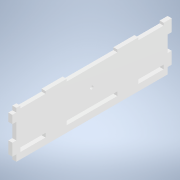
# Autodesk Inventor part: case top sides
Saved by Autodesk Inventor 2022 (Build 260153000, 153)
## iProperties
Created: 2021-05-28
Part Number: case top sides
Material: ABS Plastic
Document SubType Name: Modeling
Designer: benka
Density: 1.06 g/cm^3
Appearance: Smooth - White
Author: benka
Autodesk Inventor part; units mm, degrees
ref_plane "YZ Plane" through (0, 0, 0) normal (1, 0, 0) x (0, 1, 0)
ref_plane "XZ Plane" through (0, 0, 0) normal (0, 1, 0) x (-1, 0, 0)
ref_plane "XY Plane" through (0, 0, 0) normal (0, 0, 1) x (1, 0, 0)
sketch "Sketch1" plane through (0, 0, 0) normal (1, 0, 0) x (0, 1, 0)
  circle A0 centre (0, 0) radius 2
  line L0 (-20.007, 88.601) -> (-20.007, 57.351) projected
  line L1 (-20.007, 57.351) -> (-25.007, 57.351) projected
  line L2 (-25.007, 88.601) -> (-25.007, 57.351) projected
  line L3 (-20.007, 88.601) -> (-25.007, 88.601) projected
  line L4 (-20.007, 31.101) -> (-20.007, -31.899) projected
  line L5 (-20.007, -31.899) -> (-25.007, -31.899) projected
  line L6 (-25.007, 31.101) -> (-25.007, -31.899) projected
  line L7 (-20.007, 31.101) -> (-25.007, 31.101) projected
  line L8 (-20.007, -58.149) -> (-20.007, -89.399) projected
  line L9 (-20.007, -89.399) -> (-25.007, -89.399) projected
  line L10 (-25.007, -58.149) -> (-25.007, -89.399) projected
  line L11 (-20.007, -58.149) -> (-25.007, -58.149) projected
  line L12 (19.993, 93.601) -> (19.993, 98.601)
  line L13 (19.993, 98.601) -> (9.9915, 98.601) projected
  line L14 (9.9915, 93.601) -> (9.9915, 98.601) projected
  line L15 (-10.0085, 93.601) -> (-10.0085, 98.601) projected
  line L16 (-25.0077, 98.601) -> (-10.0085, 98.601) projected
  line L17 (-25.007, 93.601) -> (-25.007, 98.601) projected
  line L18 (-25.007, 93.601) -> (-33.007, 93.601)
  line L19 (-33.007, 93.601) -> (-33.007, -94.399)
  line L20 (-10.0085, 93.601) -> (9.9915, 93.601)
  line L21 (24.993, -99.399) -> (24.993, -94.399)
  line L22 (9.993, -99.399) -> (24.993, -99.399) projected
  line L23 (9.993, -99.399) -> (9.993, -94.399) projected
  line L24 (-10.0077, -94.399) -> (9.993, -94.399) projected
  line L25 (-10.0077, -99.399) -> (-10.0077, -94.399) projected
  line L26 (-25.0077, -99.399) -> (-10.0077, -99.399) projected
  line L27 (-25.0077, -99.399) -> (-25.0077, -94.399) projected
  line L28 (-33.0079, -94.399) -> (-25.0077, -94.399) projected
  line L29 (19.993, 93.601) -> (24.993, 93.601)
  line L30 (24.993, -94.399) -> (24.993, -89.399)
  line L31 (21.993, -89.399) -> (24.993, -89.399)
  line L32 (21.993, -89.399) -> (21.993, -58.149)
  line L33 (21.993, -58.149) -> (24.993, -58.149)
  line L34 (24.993, -58.149) -> (24.993, -31.899)
  line L35 (21.993, -31.899) -> (24.993, -31.899)
  line L36 (21.993, -31.899) -> (21.993, 31.101)
  line L37 (21.993, 31.101) -> (24.993, 31.101)
  line L38 (24.993, 31.101) -> (24.993, 57.351)
  line L39 (21.993, 57.351) -> (24.993, 57.351)
  line L40 (21.993, 57.351) -> (21.993, 88.601)
  line L41 (21.993, 88.601) -> (24.993, 88.601)
  line L42 (24.993, 88.601) -> (24.993, 93.601)
  point P0 (-29.9123, 87.1698)
  dimension "d24" = 4
  dimension "d25" = 8
  dimension "d27" = 198
  dimension "d30" = 5
  dimension "d31" = 188
  dimension "d32" = 188
  dimension "d33" = 58
  dimension "d35" = 3
  constraints: 38 end point, 6 collinear, 2 horizontal, 1 centre point, 1 vertical, 1 other
  measures "d24" diameter of A0
  measures "d25" distance of L17.start L18.end
  measures "d27" distance between parallel lines of L22 L13
  measures "d30" distance of L12.start L12.end
  measures "d31" vertical distance of L21.end L12.start
  measures "d32" distance of L18.end L19.end
  measures "d33" distance between parallel lines of L34 L19
  measures "d35" distance between parallel lines of L36 L38
extrude "Extrusion1" add sketch "Sketch1" along normal blind 5
body "Solid1"
